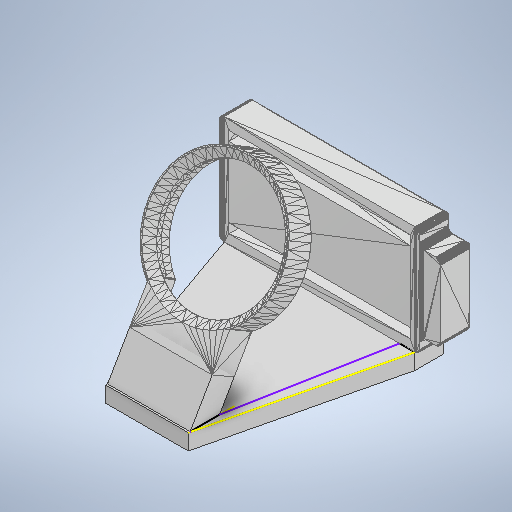
# Autodesk Inventor part: esp32-s3-devkitc-1 ChipUp PinsExposed Bottom (1)
Saved by Autodesk Inventor 2025.1 (Build 291241000, 241)
## iProperties
Created: 2025-10-02
Part Number: esp32-s3-devkitc-1 ChipUp PinsExposed Bottom (1)
Material: Generic
Document SubType Name: Modeling
Designer: Luke Buonanno
Density: 1 g/cm^3
Appearance: Default
Author: Luke Buonanno
Autodesk Inventor part; units mm, degrees
ref_plane "YZ Plane" through (0, 0, 0) normal (1, 0, 0) x (0, 1, 0)
ref_plane "XZ Plane" through (0, 0, 0) normal (0, 1, 0) x (-1, 0, 0)
ref_plane "XY Plane" through (0, 0, 0) normal (0, 0, 1) x (1, 0, 0)
sketch "Sketch1" plane through (-330.2, 304.8, 1412.4013) normal (0, -0.866, 0.5) x (1, 0, 0)
  line L0 (0.1333, -203.1273) -> (0, 0)
  line L1 (0, 0) -> (660.4052, 0)
  line L2 (660.4052, 0) -> (660.4052, -203.1273)
  line L3 (660.4052, -203.1273) -> (0.1333, -203.1273)
  point P0 (330.2, -1375.5753)
  constraints: 8 end point, 2 perpendicular, 1 horizontal
extrude "Extrusion1" add sketch "Sketch1" along normal blind 381
sketch "Sketch2" plane through (679.7379, 0, 139.7) normal (0, -1, 0) x (1, 0, 0)
  line L0 (-1.1909, -227.7462) -> (-1526.5875, -227.7462)
  line L1 (-1526.5875, -227.7462) -> (-1526.5875, -0.9438)
  line L2 (-1009.938, 1272.7013) -> (-1009.938, 1463.2013) projected
  line L3 (-1526.5875, -0.9438) -> (-1009.938, 1463.2013)
  line L4 (-349.5327, 1287.2879) -> (-349.5327, 1463.2013) projected
  line L5 (-1009.938, 1463.2013) -> (-349.5327, 1463.2013)
  line L6 (-349.5327, 1463.2013) -> (-1.1909, 0)
  line L7 (-1.1909, 0) -> (-1.1909, -227.7462)
  point P0 (-679.7379, -139.7)
  constraints: 12 end point, 3 perpendicular, 1 horizontal
extrude "Extrusion2" add sketch "Sketch2" along normal blind 127
sketch "Sketch3" plane through (679.7379, 0, 139.7) normal (0, 1, 0) x (1, 0, 0)
  line L0 (-1.1909, 0) -> (-349.5327, -1463.2013) projected
  line L1 (-346.1567, -1449.0205) -> (-1.1909, 0)
  line L2 (-1.1909, 0) -> (-123.0131, 0)
  line L3 (-349.5327, -1096.7879) -> (-349.5327, -1214.1265) projected
  line L4 (-123.0131, 0) -> (-349.5327, -1214.1265)
  line L5 (-349.5327, -1214.1265) -> (-349.5327, -1449.0205)
  line L6 (-349.5327, -1449.0205) -> (-346.1567, -1449.0205)
  point P0 (-679.7379, 139.7)
  constraints: 10 end point, 2 perpendicular, 1 collinear, 1 horizontal, 1 point on line
body "Solid1"
